3a7386d9-e6da-4163-999a-5fb095b64bfa (Autodesk Fusion 360 design; units mm, degrees)
Autodesk Fusion 360 part; units mm, degrees
sketch "Sketch1" plane through (0, 0, 0) normal (0, 0, 1) x (1, 0, 0)
  circle A0 centre (0, 0) radius 3.175
  circle A1 centre (0, 0) radius 4.7625
  dimension "d1" = 6.35
  dimension "d2" = 9.525
  measures "d1" diameter of A0
  measures "d2" diameter of A1
extrude "Extrude1" add sketch "Sketch1" along normal blind 9.525
sketch "Sketch2" plane through (0, 0, 0) normal (0, 0, -1) x (-1, 0, 0)
  circle A0 centre (0, 0) radius 4.7625
  circle A1 centre (0, 0) radius 6.35
  circle A2 centre (0, 0) radius 3.175
  dimension "d5" = 12.7
  measures "d5" diameter of A1
extrude "Extrude2" add sketch "Sketch2" against normal blind 1.5875 contours A1
equation "d1 = Shaft_ID"
equation "d2 = Housing_ID"
equation "d3 = Length"
equation "d5 = Flange_OD"
equation "d6 = FlangeT"
equation "Shaft_ID = ( 1 / 4 ) * 1 in"
equation "Housing_ID = ( 3 / 8 ) * 1 in"
equation "FlangeT = ( -1 / 16 ) * 1 in"
equation "Length = ( 3 / 8 ) * 1 in"
equation "Flange_OD = ( 1 / 2 ) * 1 in"
